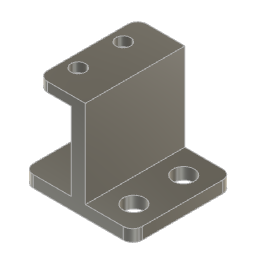
Microswitch Limit Mount v1 (Autodesk Fusion 360 design; units mm, degrees)
Autodesk Fusion 360 part; units mm, degrees
note: some values were not read from the file. Set by a fixed rule: which sketch regions a step uses.
sketch "Sketch1" plane through (0, 0, 0) normal (0, 0, 1) x (1, 0, 0)
  line L0 (5, 10.5) -> (-5, 10.5)
  line L1 (-5, 10.5) -> (-5, -10.5)
  line L2 (-5, -10.5) -> (5, -10.5)
  line L3 (5, -10.5) -> (5, 10.5)
  line L4 (5, 10.5) -> (-5, -10.5) construction
  line L5 (-5, 10.5) -> (5, -10.5) construction
  line L6 (5, -4.75) -> (-5, -4.75)
  line L7 (-5, -4.75) -> (-5, 4.75)
  line L8 (-5, 4.75) -> (5, 4.75)
  line L9 (5, 4.75) -> (5, -4.75)
  line L10 (5, -4.75) -> (-5, 4.75) construction
  line L11 (-5, -4.75) -> (5, 4.75) construction
  circle A0 centre (-2.2619, 4.75) radius 1.55
  circle A1 centre (-2.2619, -4.75) radius 1.55
  line L12 (5, 10.5) -> (2, 10.5)
  line L13 (2, 10.5) -> (2, -10.5)
  line L14 (2, -10.5) -> (5, -10.5)
  line L15 (5, -10.5) -> (5, 10.5)
  dimension "d1" = 10
  dimension "d2" = 21
  dimension "d3" = 10
  dimension "d4" = 9.5
  dimension "d5" = 3.1
  dimension "d6" = 3.1
  dimension "d7" = 3
  constraint horizontal L0
  constraint perpendicular L0 L1
  constraint parallel L0 L2
  constraint parallel L1 L3
  constraint coincident L4 origin
  constraint coincident L5 origin
  constraint horizontal L6
  constraint perpendicular L6 L7
  constraint parallel L6 L8
  constraint parallel L7 L9
  constraint coincident L10 origin
  constraint coincident L11 origin
  constraint coincident L8 A0.centre
  constraint coincident L5 A0.centre
  constraint coincident L4 A1.centre
  constraint coincident L6 A1.centre
  constraint horizontal L12
  constraint vertical L13
  constraint horizontal L14
  constraint vertical L15
  measures "d1" distance of L1.end L2.end
  measures "d2" distance of L0.end L1.end
  measures "d3" distance of L7.end L8.end
  measures "d4" distance of L6.end L7.end
  measures "d5" diameter of A0
  measures "d6" diameter of A1
  measures "d7" distance of L0.start L12.end
extrude "Extrude1" add sketch "Sketch1" along normal blind 2 contours L0 L3 L8 L12 L13 L15 | L0 L1 L8 A0 L13 | L3 L6 L8 L9 L13 L15 | L1 L6 L7 L8 A0 A1 L13 | L2 L3 L6 L13 L14 L15 | L1 L2 L6 A1 L13
extrude "Extrude2" add sketch "Sketch1" against normal blind 19 contours L0 L3 L8 L12 L13 L15 | L3 L6 L8 L9 L13 L15 | L2 L3 L6 L13 L14 L15
sketch "Sketch2" plane through (5, 0, 0) normal (1, 0, 0) x (0, 1, 0)
  line L0 (10.5, -19) -> (10.5, 2)
  line L1 (10.5, 2) -> (-10.5, 2)
  line L2 (-10.5, 2) -> (-10.5, -19)
  line L3 (-10.5, -19) -> (10.5, -19)
  line L4 (-10.5, -19) -> (10.5, -19)
  line L5 (10.5, -19) -> (10.5, -16.5)
  line L6 (10.5, -16.5) -> (-10.5, -16.5)
  line L7 (-10.5, -16.5) -> (-10.5, -19)
  dimension "d12" = 2.5
  constraint horizontal L4
  constraint vertical L5
  constraint horizontal L6
  constraint vertical L7
  constraint coincident L2.end L3.start
  measures "d12" distance of L2.end L6.end
extrude "Extrude3" add sketch "Sketch2" along normal blind 10 and the other way blind 13 contours L0 L2 L3 L4 L5 L6 L7
sketch "Sketch3" plane through (0, 0, -16.5) normal (0, 0, 1) x (-1, 0, 0)
  line L0 (-5, -10.5) -> (-5, 10.5)
  line L1 (-5, 10.5) -> (-15, 10.5)
  line L2 (-15, 10.5) -> (-15, -10.5)
  line L3 (-15, -10.5) -> (-5, -10.5)
  line L4 (-10, -10.5) -> (-10, 10.5)
  line L5 (-15, 0) -> (-5, 0)
  line L6 (-10, 0) -> (-10, -10.5)
  circle A0 centre (-10, -5.25) radius 2.25
  line L7 (-10, 0) -> (-10, 10.5)
  circle A1 centre (-10, 5.25) radius 2.25
  dimension "d17" = 4.5
  dimension "d18" = 4.5
  constraint midpoint L3 L4.start
  constraint midpoint L1 L4.end
  constraint midpoint L2 L5.start
  constraint midpoint L0 L5.end
  constraint midpoint L5 L6.start
  constraint midpoint L6 A0.centre
  constraint midpoint L7 A1.centre
  measures "d17" diameter of A0
  measures "d18" diameter of A1
fillet "Fillet1" radius 2 6 edges at (15, -10.5, -17.75) (15, 10.5, -17.75) (-8, -10.5, -17.75) (-5, -10.5, 1) (-5, 10.5, 1) (-8, 10.5, -17.75)
extrude "Extrude4" cut sketch "Sketch3" against normal blind 7 contours L4 L6 A0 | L4 L6 A0 | L4 L7 A1 | L4 L7 A1
